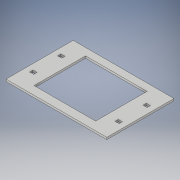
# Autodesk Inventor part: Table_plate
Saved by Autodesk Inventor 2019.4 (Build 234330000, 330)
## iProperties
Created: 2019-12-14
Part Number: Table_plate
Material: Generic
Document SubType Name: Modeling
Designer: fabfarm
Density: 1 g/cm^3
Appearance: Default
Author: fabfarm
Autodesk Inventor part; units mm, degrees
ref_plane "YZ Plane" through (0, 0, 0) normal (1, 0, 0) x (0, 1, 0)
ref_plane "XZ Plane" through (0, 0, 0) normal (0, 1, 0) x (-1, 0, 0)
ref_plane "XY Plane" through (0, 0, 0) normal (0, 0, 1) x (1, 0, 0)
sketch "Sketch1" plane through (0, 0, 0) normal (0, 1, 0) x (-1, 0, 0)
  line L0 (0, 0) -> (900, 0)
  line L1 (900, 0) -> (900, -600)
  line L2 (900, -600) -> (0, -600)
  line L3 (0, -600) -> (0, 0)
  line L4 (725, -75) -> (175, -75)
  line L5 (175, -75) -> (175, -535)
  line L6 (175, -535) -> (725, -535)
  line L7 (725, -535) -> (725, -75)
  dimension "d0" = 900
  dimension "d1" = 600
  dimension "d23" = 175
  dimension "d24" = 75
  dimension "d25" = 460
  dimension "d26" = 550
  constraints: 16 end point, 4 parallel, 2 horizontal, 2 perpendicular
  measures "d0" distance of L0.start L0.end
  measures "d1" distance between parallel lines of L0 L2
  measures "d23" distance between parallel lines of L3 L5
  measures "d24" distance between parallel lines of L0 L4
  measures "d25" distance of L4.end L5.end
  measures "d26" distance of L4.start L4.end
extrude "Extrusion4" add sketch "Sketch1" along normal blind 18.55
sketch "Sketch4" plane through (0, 18.55, 0) normal (0, 1, 0) x (1, 0, 0)
  line L0 (-850, 440) -> (-812.9, 440)
  line L1 (-812.9, 440) -> (-812.9, 410)
  line L2 (-812.9, 410) -> (-850, 410)
  line L3 (-850, 410) -> (-850, 440)
  line L4 (-850, 160) -> (-812.9, 160)
  line L5 (-812.9, 160) -> (-812.9, 190)
  line L6 (-812.9, 190) -> (-850, 190)
  line L7 (-850, 190) -> (-850, 160)
  line L8 (-87.1, 440) -> (-50, 440)
  line L9 (-50, 440) -> (-50, 410)
  line L10 (-50, 410) -> (-87.1, 410)
  line L11 (-87.1, 410) -> (-87.1, 440)
  line L12 (-87.1, 160) -> (-50, 160)
  line L13 (-50, 160) -> (-50, 190)
  line L14 (-50, 190) -> (-87.1, 190)
  line L15 (-87.1, 190) -> (-87.1, 160)
  line L16 (0, 600) -> (-900, 600) projected
  line L17 (-900, 600) -> (-900, 0) projected
  line L18 (-900, 0) -> (0, 0) projected
  line L19 (0, 0) -> (0, 600) projected
  dimension "d29" = 160
  dimension "d30" = 50
  dimension "d33" = 30
  dimension "d34" = 37.1
  dimension "d35" = 30
  dimension "d36" = 50
  dimension "d39" = 160
  constraints: 32 end point, 8 parallel, 7 point on line, 4 horizontal, 4 perpendicular, 2 collinear
  measures "d29" distance between parallel lines of L16 L0
  measures "d30" distance between parallel lines of L17 L3
  measures "d33" distance of L2.end L0.start
  measures "d34" distance of L0.start L0.end
  measures "d35" distance of L6.end L4.start
  measures "d36" distance between parallel lines of L19 L13
  measures "d39" distance between parallel lines of L18 L4
extrude "Extrusion5" cut sketch "Sketch4" against normal blind 50 contours L0 L1 L2 L3 | L7 L6 L5 L4 | L8 L9 L10 L11 | L15 L14 L13 L12
body "Solid2"
